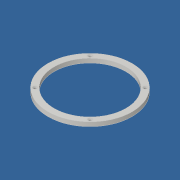
# Autodesk Inventor part: Drehkranz_B
Saved by Autodesk Inventor 2016 (Build 200138000, 138)
## iProperties
Created: 2015-09-24
Part Number: Drehkranz_B
Material: ABS-Kunststoff
Document SubType Name: Modeling
Designer: 4ndreas
Density: 1.06 g/cm^3
Appearance: Glatt - weiß
Mass: 91.4912 g
Surface Area: 296.874 cm^2
Volume: 86.3124 cm^3
Author: 4ndreas
Autodesk Inventor part; units mm, degrees
ref_plane "YZ Plane" through (0, 0, 0) normal (1, 0, 0) x (0, 1, 0)
ref_plane "XZ Plane" through (0, 0, 0) normal (0, 1, 0) x (-1, 0, 0)
ref_plane "XY Plane" through (0, 0, 0) normal (0, 0, 1) x (1, 0, 0)
sketch "Skizze1" plane through (0, 0, 0) normal (0, 0, 1) x (1, 0, 0)
  circle A0 centre (0, 0) radius 72
  circle A1 centre (0, 0) radius 101.5
  circle A2 centre (0, 0) radius 86.75
  dimension "d0" = 144
  dimension "d1" = 203
  dimension "d2" = 29.5
  dimension "d3" = 14.75
  constraints: 3 centre point, 3 coincident
  measures "d0" diameter of A0
  measures "d1" diameter of A1
  measures "d2" radial gap between concentric circles of A0 A1
  measures "d3" radial gap between concentric circles of A0 A2
extrude "Extrusion1" add sketch "Skizze1" along normal blind 10 contours A1
sketch "Skizze2" plane through (0, 0, 10) normal (0, 0, 1) x (1, 0, 0)
  line L0 (-66.5564, -66.5564) -> (66.5564, -66.5564)
  line L1 (66.5564, -66.5564) -> (66.5564, 66.5564)
  line L2 (66.5564, 66.5564) -> (-66.5564, 66.5564)
  line L3 (-66.5564, 66.5564) -> (-66.5564, -66.5564)
  line L4 (-66.5564, -66.5564) -> (66.5564, 66.5564) construction
  line L5 (66.5564, -66.5564) -> (-66.5564, 66.5564) construction
  circle A0 centre (0, 0) radius 94.125 construction
  circle A1 centre (0, 0) radius 86.75 construction
  circle A2 centre (0, 0) radius 101.5 construction
  dimension "d15" = 14.75
  dimension "d16" = 7.375
  constraints: 12 end point, 4 coincident, 2 midpoint, 2 parallel, 2 perpendicular, 1 horizontal, 3 other
  measures "d15" radial gap between concentric circles of A1 A2
hole "Bohrung1" at (-66.5564, 66.5564, 10) at (66.5564, 66.5564, 10) at (66.5564, -66.5564, 10) at (-66.5564, -66.5564, 10) direction (0, 0, -1) diameter 4.9 end through all countersink diameter 9 countersink angle 90
equation "\"d3\" = 0.5 * d2"
equation "\"d16\" = 0.5 * d15"
